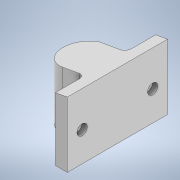
# Autodesk Inventor part: backcover_clamp_NEW
Saved by Autodesk Inventor 2020 (Build 240168000, 168)
## iProperties
Created: 2019-07-30
Part Number: backcover_clamp_NEW
Material: Generic
Document SubType Name: Modeling
Designer: erwin
Density: 1 g/cm^3
Appearance: Default
Author: erwin
Autodesk Inventor part; units mm, degrees
ref_plane "YZ Plane" through (0, 0, 0) normal (1, 0, 0) x (0, 1, 0)
ref_plane "XZ Plane" through (0, 0, 0) normal (0, 1, 0) x (-1, 0, 0)
ref_plane "XY Plane" through (0, 0, 0) normal (0, 0, 1) x (1, 0, 0)
sketch "Sketch1" plane through (0, 0, 0) normal (0, 1, 0) x (-1, 0, 0)
  line L0 (-2.536256, 16.837397) -> (1.463744, 16.837397)
  line L1 (1.463744, -17) -> (-2.536256, -17)
  line L2 (-2.536256, -17) -> (-2.536256, 16.837397)
  circle A0 centre (8.963744, -0.162603) radius 4.5
  arc A1 (10.463744, -7) -> (8.963744, 6.837397) centre (8.963744, -0.162603) ccw
  line L3 (8.963744, 6.837397) -> (3.463744, 6.837397)
  line L4 (10.463744, -7) -> (3.463744, -7)
  line L5 (1.463744, 16.837397) -> (1.463744, 8.837397)
  line L6 (1.463744, -9) -> (1.463744, -17)
  arc A2 (1.463744, 8.837397) -> (3.463744, 6.837397) centre (3.463744, 8.837397) ccw
  arc A3 (3.463744, -7) -> (1.463744, -9) centre (3.463744, -9) ccw
  point P0 (0, 0)
  point P1 (1.463744, 6.837397)
  point P2 (1.463744, -7)
  dimension "d0" = 9
  dimension "d1" = 2.5
  dimension "d2" = 11.5
  dimension "d3" = 4
  dimension "d4" = 4
  dimension "d5" = 10
  dimension "d6" = 10
  dimension "d7" = 2
  constraints: 14 end point, 6 perpendicular, 6 point on circle, 4 centre point, 4 point on line, 4 tangent, 3 parallel, 1 equal radius, 1 horizontal
  measures "d0" diameter of A0
  measures "d1" radial gap between concentric circles of A0 A1
  measures "d2" distance from line of L2 A0.centre
  measures "d3" distance between parallel lines of L6 L2
  measures "d4" distance between parallel lines of L2 L5
  measures "d5" distance of point (1.464, -7) L1.start
  measures "d6" distance of L0.end point (1.464, 6.837)
  measures "d7" radius of A2
extrude "Extrusion1" add sketch "Sketch1" along normal blind 20
sketch "Sketch2" plane through (0, 20, 0) normal (0, 1, 0) x (1, 0, 0)
  circle A0 centre (-8.963744, 0.162603) radius 4.5
  point P0 (0, 0)
extrude "Extrusion2" add sketch "Sketch2" against normal blind 3
sketch "Sketch3" plane through (-1.463744, 0, -17) normal (-1, 0, 0) x (0, 0, 1)
  line L0 (0, 0) -> (8, 0)
  line L1 (25.837397, 0) -> (33.837397, 0)
  line L2 (0, 0) -> (0, 20)
  line L3 (33.837397, 0) -> (33.837397, 20)
  point P0 (17, 0)
  point P1 (5, 10)
  point P2 (28.837397, 10)
  dimension "d13" = 10
  dimension "d14" = 10
  dimension "d15" = 5
  dimension "d16" = 5
  measures "d13" distance from line of L0 point (5, 10)
  measures "d14" distance from line of L1 point (28.837, 10)
  measures "d15" distance from line of L2 point (5, 10)
  measures "d16" distance from line of L3 point (28.837, 10)
hole "Hole1" at (-1.463744, 10, -12) at (-1.463744, 10, 11.837397) direction (1, 0, 0) diameter 3.5 end through all countersink diameter 8 countersink angle 90
draft "FaceDraft1" angle 10 pull direction (-1, 0, 0) faces at (1.186208, 20, 2.743251) fixed edges at (2.536256, 20, -0.081301)
move faces "Move1" translate (-0.347296, 1.969616, 0) faces at (1.184502, 19.761649, -2.898571)
equation "\"d3\" = d4"
equation "\"d6\" = d5"
equation "\"d14\" = d13"
equation "\"d16\" = d15"
body "Solid1"
